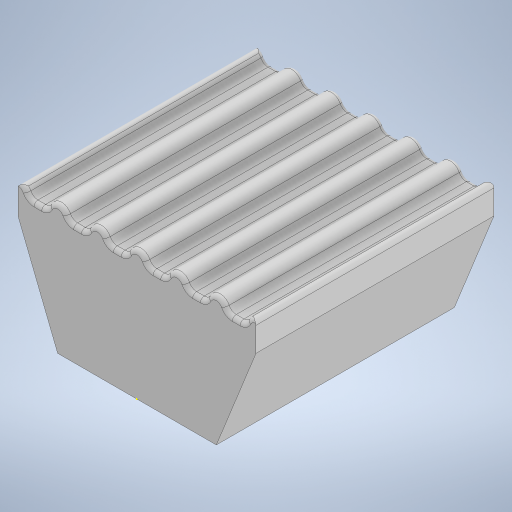
# Autodesk Inventor part: Top
Saved by Autodesk Inventor 2024 (Build 280153000, 153)
## iProperties
Created: 2024-03-28
Part Number: Top
Material: Generic
Document SubType Name: Modeling
Designer: t60147996
Density: 1 g/cm^3
Appearance: Default
Author: t60147996
Autodesk Inventor part; units mm, degrees
ref_plane "YZ Plane" through (0, 0, 0) normal (1, 0, 0) x (0, 1, 0)
ref_plane "XZ Plane" through (0, 0, 0) normal (0, 1, 0) x (-1, 0, 0)
ref_plane "XY Plane" through (0, 0, 0) normal (0, 0, 1) x (1, 0, 0)
sketch "Sketch1" plane through (0, 0, 0) normal (0, 1, 0) x (-1, 0, 0)
  line L0 (-25.4, 38.1) -> (25.4, 38.1)
  line L1 (25.4, 38.1) -> (25.4, -38.1)
  line L2 (25.4, -38.1) -> (-25.4, -38.1)
  line L3 (-25.4, -38.1) -> (-25.4, 38.1)
  line L4 (-25.4, 38.1) -> (25.4, -38.1) construction
  line L5 (25.4, 38.1) -> (-25.4, -38.1) construction
  point P0 (0, 0)
  dimension "d0" = 50.8
  dimension "d1" = 76.2
  constraints: 12 end point, 2 midpoint, 2 parallel, 1 horizontal, 1 perpendicular
  measures "d0" distance of L1.end L2.end
  measures "d1" distance of L0.end L1.end
extrude "Extrusion1" add sketch "Sketch1" along normal blind 38.1
sketch "Sketch2" plane through (25.4, 0, -38.1) normal (0, 0, -1) x (-1, 0, 0)
  line L0 (0, 0) -> (0, 38.1) projected
  line L1 (0, 38.1) -> (-12.7, 38.1)
  line L2 (-12.7, 38.1) -> (-12.7, 31.75)
  line L3 (-12.7, 31.75) -> (0, 31.75)
  line L4 (0, 31.75) -> (0, 38.1)
  line L5 (0, 38.1) -> (50.8, 38.1) projected
  line L6 (50.8, 38.1) -> (63.5, 38.1)
  line L7 (63.5, 38.1) -> (63.5, 31.75)
  line L8 (63.5, 31.75) -> (50.8, 31.75)
  line L9 (50.8, 31.75) -> (50.8, 38.1)
  line L10 (0, 0) -> (50.8, 0) projected
  line L11 (63.5, 31.75) -> (50.8, 0)
  line L12 (-12.7, 31.75) -> (0, 0)
  line L13 (0, 31.75) -> (0, 0)
  line L14 (50.8, 31.75) -> (50.8, 0)
  point P0 (25.4, 0)
  dimension "d4" = 12.7
  dimension "d5" = 6.35
  dimension "d6" = 12.7
  constraints: 24 end point, 5 parallel, 2 horizontal, 2 perpendicular, 1 collinear, 1 point on line
  measures "d4" distance of L3.end L2.end
  measures "d5" distance of L2.end L1.end
  measures "d6" distance of L7.end L8.end
extrude "Extrusion2" add sketch "Sketch2" against normal up to surface (76.2 mm away) contours L12 L3 L0 | L3 L2 L1 L0 | L14 L8 L11 | L8 L9 L6 L7
sketch "Sketch3" plane through (38.1, 38.1, -38.1) normal (0, 0, -1) x (-1, 0, 0)
  line L0 (76.2, 0) -> (0, 0) projected
  circle A0 centre (0, 0) radius 3.175
  circle A1 centre (12.7, 0) radius 3.175
  circle A2 centre (25.4, 0) radius 3.175
  circle A3 centre (38.1, 0) radius 3.175
  circle A4 centre (50.8, 0) radius 3.175
  circle A5 centre (63.5, 0) radius 3.175
  circle A6 centre (76.2, 0) radius 3.175
  point P0 (38.1, -38.1)
  dimension "d9" = 6.35
  dimension "d10" = 6.35
  dimension "d11" = 6.35
  dimension "d12" = 6.35
  dimension "d13" = 6.35
  dimension "d14" = 6.35
  dimension "d15" = 6.35
  constraints: 7 centre point
  measures "d9" diameter of A0
  measures "d10" diameter of A1
  measures "d11" diameter of A2
  measures "d12" diameter of A3
  measures "d13" diameter of A4
  measures "d14" diameter of A5
  measures "d15" diameter of A6
extrude "Extrusion3" add sketch "Sketch3" against normal up to surface (76.2 mm away)
sketch "Sketch4" plane through (25.4, 0, -38.1) normal (0, 0, -1) x (-1, 0, 0)
  arc A0 (-9.525, 38.1) -> (-12.7, 34.925) centre (-12.7, 38.1) ccw projected
  line L0 (-12.7, 41.275) -> (-12.7, 34.925)
  point P0 (25.4, 0)
  constraints: 2 end point, 1 point on circle, 1 vertical
extrude "Extrusion4" cut sketch "Sketch4" against normal through all
sketch "Sketch5" plane through (25.4, 0, -38.1) normal (0, 0, -1) x (-1, 0, 0)
  arc A0 (63.5, 34.925) -> (60.325, 38.1) centre (63.5, 38.1) ccw projected
  line L0 (63.5, 34.925) -> (63.5, 41.275)
  point P0 (25.4, 0)
  constraints: 2 end point, 1 point on circle, 1 vertical
extrude "Extrusion5" cut sketch "Sketch5" against normal through all
fillet "Fillet1" radius 2.54 12 edges at (34.925, 38.1, 0) (28.575, 38.1, 0) (22.225, 38.1, 0) (15.875, 38.1, 0) (9.525, 38.1, 0) (3.175, 38.1, 0) (-3.175, 38.1, 0) (-9.525, 38.1, 0) (-15.875, 38.1, 0) (-22.225, 38.1, 0) (-28.575, 38.1, 0) (-34.925, 38.1, 0)
fillet "Fillet2" radius 1.27 52 edges at (-38.1, 41.275, 0) (-34.3192, 38.4814, 38.1) (-31.75, 38.1, 38.1) (-29.1808, 38.4814, 38.1) (-25.4, 41.275, 38.1) (-21.6192, 38.4814, 38.1) (-19.05, 38.1, 38.1) (-16.4808, 38.4814, 38.1) (-12.7, 41.275, 38.1) (-8.9192, 38.4814, 38.1) (-6.35, 38.1, 38.1) (-3.7808, 38.4814, 38.1) (0, 41.275, 38.1) (3.7808, 38.4814, 38.1) (6.35, 38.1, 38.1) (8.9192, 38.4814, 38.1) (12.7, 41.275, 38.1) (16.4808, 38.4814, 38.1) (19.05, 38.1, 38.1) (21.6192, 38.4814, 38.1) (25.4, 41.275, 38.1) (29.1808, 38.4814, 38.1) (31.75, 38.1, 38.1) (34.3192, 38.4814, 38.1) (36.4266, 40.7982, 38.1) (-36.4266, 40.7982, 38.1) (38.1, 41.275, 0) (29.1808, 38.4814, -38.1) (31.75, 38.1, -38.1) (34.3192, 38.4814, -38.1) (36.4266, 40.7982, -38.1) (21.6192, 38.4814, -38.1) (19.05, 38.1, -38.1) (16.4808, 38.4814, -38.1) (12.7, 41.275, -38.1) (8.9192, 38.4814, -38.1) (6.35, 38.1, -38.1) (3.7808, 38.4814, -38.1) (0, 41.275, -38.1) (-3.7808, 38.4814, -38.1) (-6.35, 38.1, -38.1) (-8.9192, 38.4814, -38.1) (-12.7, 41.275, -38.1) (-16.4808, 38.4814, -38.1) (-19.05, 38.1, -38.1) (-21.6192, 38.4814, -38.1) (-25.4, 41.275, -38.1) (-29.1808, 38.4814, -38.1) (-31.75, 38.1, -38.1) (-34.3192, 38.4814, -38.1) (-36.4266, 40.7982, -38.1) (25.4, 41.275, -38.1)
sketch "Sketch6" plane through (-25.4, 0, 38.1) normal (0, 0, 1) x (1, 0, 0)
  point P0 (25.4, 0)
body "Solid1"
